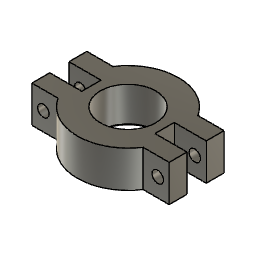
bearing_holder v1 (Autodesk Fusion 360 design; units mm, degrees)
Autodesk Fusion 360 part; units mm, degrees
sketch "Sketch1" plane through (0, 0, 0) normal (0, 0, 1) x (1, 0, 0)
  circle A0 centre (0, 0) radius 6.05
  circle A1 centre (0, 0) radius 11.05
  line L0 (15, 6) -> (-15, 6)
  line L1 (-15, 6) -> (-15, -6)
  line L2 (-15, -6) -> (15, -6)
  line L3 (15, -6) -> (15, 6)
  line L4 (15, 6) -> (-15, -6) construction
  line L5 (-15, 6) -> (15, -6) construction
  dimension "d2" = 12.1
  dimension "d3" = 5
  dimension "d4" = 30
  dimension "d5" = 12
  constraint coincident A0.centre A1.centre
  constraint horizontal L0
  constraint perpendicular L0 L1
  constraint parallel L0 L2
  constraint parallel L1 L3
  constraint coincident L4 A0.centre
  constraint coincident L5 A0.centre
  measures "d2" diameter of A0
  measures "d3" distance of A0 A1
  measures "d4" distance of L0.start L0.end
  measures "d5" distance of L0.start L2.end
extrude "Extrude1" add sketch "Sketch1" along normal blind 8 contours A0 A1 L0 L2 | A0 A1 L0 | A0 A1 L2 | A0 A1 L0 L2 | A1 L0 L2 L3 | A1 L0 L1 L2
sketch "Sketch2" plane through (0, -6, 0) normal (0, -1, 0) x (1, 0, 0)
  line L0 (9.2791, 0) -> (15, 0)
  line L1 (15, 0) -> (15, 8)
  line L2 (15, 8) -> (9.2791, 8)
  line L3 (9.2791, 8) -> (9.2791, 0)
  circle A0 centre (12.5, 4) radius 1.25
  circle A1 centre (-12.5, 4) radius 1.25
  line L4 (12.5, 4) -> (-12.5, 4) construction
  line L5 (9.2791, 8) -> (-9.2791, 8)
  line L6 (0, 0) -> (0, 4) construction
  dimension "d8" = 2.5
  dimension "d9" = 2.5
  dimension "d10" = 4
  dimension "d11" = 25
  constraint coincident A0.centre L4.start
  constraint coincident A1.centre L4.end
  constraint coincident L6.start origin
  constraint midpoint L4 L6.end
  constraint perpendicular L4 L6
  measures "d8" diameter of A0
  measures "d9" diameter of A1
  measures "d10" distance of L4 L5
  measures "d11" distance of A0.centre A1.centre
extrude "Extrude2" cut sketch "Sketch2" against normal blind 12 contours A0 | A1
sketch "Sketch3" plane through (0, 0, 8) normal (0, 0, 1) x (-1, 0, 0)
  circle A0 centre (0, 0) radius 6.05
  line L0 (-15, 6) -> (-15, -6)
  line L1 (-15, -6) -> (-9.2791, -6)
  arc A1 (-9.2791, -6) -> (9.2791, -6) centre (0, 0) ccw
  line L2 (9.2791, -6) -> (15, -6)
  line L3 (15, -6) -> (15, 6)
  line L4 (15, 6) -> (9.2791, 6)
  arc A2 (9.2791, 6) -> (-9.2791, 6) centre (0, 0) ccw
  line L5 (-9.2791, 6) -> (-15, 6)
  line L6 (-15, 2.1) -> (-8, 2.1)
  line L7 (-8, 2.1) -> (-8, -2.1)
  line L8 (-8, -2.1) -> (-15, -2.1)
  line L9 (-15, -2.1) -> (-15, 2.1)
  line L10 (0, 0) -> (0, 0.3641)
  line L11 (0, 0.3641) -> (0, 11.05)
  line L12 (0, 0) -> (-6.05, 0)
  line L13 (15, 2.1) -> (8, 2.1)
  line L14 (15, -2.1) -> (15, 2.1)
  line L15 (8, -2.1) -> (15, -2.1)
  line L16 (8, 2.1) -> (8, -2.1)
  dimension "d14" = 4.2
  dimension "d15" = 8
  constraint horizontal L6
  constraint vertical L7
  constraint horizontal L8
  constraint vertical L9
  constraint coincident A0.centre A1.centre
  constraint vertical L10
  constraint midpoint A2 L11.end
  constraint parallel L10 L11
  constraint coincident A0 L12.end
  constraint perpendicular L10 L12
  constraint symmetric L6 L8 L12
  constraint collinear L0 L9
  constraint symmetric L6.start L11 L13.start
  constraint symmetric L6.end L11 L13.end
  constraint symmetric L7.end L11 L15.start
  constraint symmetric L8.end L11 L14.start
  measures "d14" distance of L6.start L8.end
  measures "d15" distance of A0.centre L7
extrude "Extrude3" cut sketch "Sketch3" against normal blind 8 contours L0 L6 L7 L8 L9 | L3 L13 L14 L15 L16
chamfer "Chamfer1" distance 0.5 angle 45 1 edges at (-5.6406, 2.1878, 0)
equation "bearing_hole = 12.1 mm"
equation "d2 = bearing_hole"
